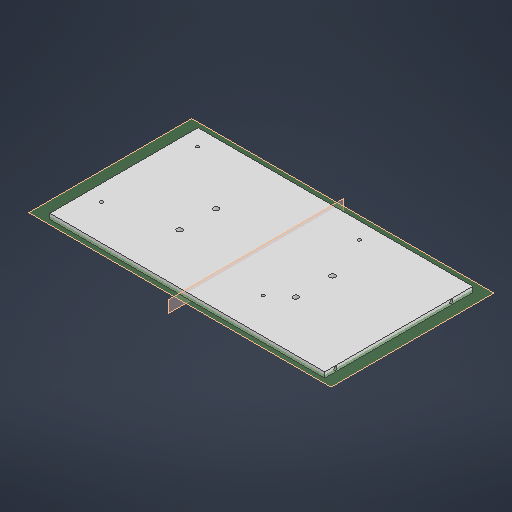
# Autodesk Inventor part: midplate
Saved by Autodesk Inventor 2025.1 (Build 291241000, 241)
## iProperties
Created: 2025-03-19
Part Number: midplate
Material: Generic
Document SubType Name: Modeling
Designer: m_kni
Density: 1 g/cm^3
Appearance: Default
Author: m_kni
Autodesk Inventor part; units mm, degrees
ref_plane "YZ Plane" through (0, 0, 0) normal (1, 0, 0) x (0, 1, 0)
ref_plane "XZ Plane" through (0, 0, 0) normal (0, 1, 0) x (-1, 0, 0)
ref_plane "XY Plane" through (0, 0, 0) normal (0, 0, 1) x (1, 0, 0)
sketch "Sketch1" plane through (0, 0, 0) normal (0, 1, 0) x (-1, 0, 0)
  circle A0 centre (-37.3734, -58.1709) radius 1.5
  circle A1 centre (112.6266, 30.8291) radius 1.5
  circle A2 centre (-37.3734, 30.8291) radius 1.5
  circle A3 centre (112.6266, -58.1709) radius 1.5
  circle A4 centre (54.1266, -16.9209) radius 2.5
  circle A5 centre (-53.8734, 17.0791) radius 2.5
  circle A6 centre (54.1266, 17.0791) radius 2.5
  circle A7 centre (-53.8734, -16.9209) radius 2.5
  line L0 (-127.3734, 73.8291) -> (127.6266, 73.8291)
  line L1 (-127.3734, -73.6709) -> (-127.3734, 73.8291)
  line L2 (127.6266, -73.6709) -> (-127.3734, -73.6709)
  line L3 (127.6266, 73.8291) -> (127.6266, -73.6709)
  point P0 (0, 0)
  point P1 (0.1266, 73.8291)
  constraints: 8 centre point, 8 end point
extrude "Extrusion1" add sketch "Sketch1" along normal blind 10
sketch "Sketch2" plane through (127.3734, 0, 73.8291) normal (1, 0, 0) x (0, 0, -1)
  line L0 (147.5, 0) -> (147.5, 10) projected
  line L1 (0, 0) -> (0, 10) projected
  circle A0 centre (127.5, 5) radius 1.5
  circle A1 centre (20, 5) radius 1.5
  point P0 (73.8291, 0)
  point P1 (0, 5)
  dimension "d2" = 20
  dimension "d3" = 20
  dimension "d4" = 3
  dimension "d5" = 3
  constraints: 2 centre point, 2 coincident, 1 midpoint
  measures "d2" distance from line of point (127.5, 5) L0
  measures "d3" distance of point (20, 5) point (0, 5)
  measures "d4" diameter of A0
  measures "d5" diameter of A1
extrude "Extrusion2" cut sketch "Sketch2" against normal blind 6
ref_plane "Work Plane1" through (-0.1266, 0, 73.8291) normal (1, 0, 0) x (0, 0, -1)
mirror "Mirror1" about plane through (-0.1266, 0, 73.8291) normal (1, 0, 0) of "Extrusion2"
sketch "Sketch3" plane through (-127.6266, 0, 73.8291) normal (0, 0, 1) x (1, 0, 0)
  line L0 (255, 10) -> (0, 10) projected
  line L1 (255, 0) -> (0, 0)
  line L2 (0, 0) -> (0, 10)
  line L3 (0, 10) -> (255, 10)
  line L4 (255, 10) -> (255, 0)
  point P0 (127.6266, 0)
  constraints: 8 end point, 2 parallel, 1 horizontal, 1 perpendicular
extrude "Extrusion3" cut sketch "Sketch3" against normal blind 10
sketch "Sketch4" plane through (0, 10, 0) normal (0, 1, 0) x (1, 0, 0)
  line L0 (127.3734, -63.8291) -> (127.3734, 73.6709) projected
  line L1 (-127.6266, -63.8291) -> (127.3734, -63.8291)
  line L2 (127.3734, -63.8291) -> (127.3734, 73.6709)
  line L3 (127.3734, 73.6709) -> (-127.6266, 73.6709)
  line L4 (-127.6266, 73.6709) -> (-127.6266, -63.8291)
  point P0 (0, 0)
  constraints: 8 end point, 2 parallel, 1 horizontal, 1 perpendicular
ref_plane "Work Plane2" through (0, 5, 0) normal (0, 1, 0) x (1, 0, 0)
extrude "Extrusion4" cut sketch "Sketch4" against normal blind 2.5
mirror "Mirror2" about plane through (0, 5, 0) normal (0, 1, 0) of "Extrusion4"
ref_plane "Work Plane3" through (0, 5, 0) normal (0, 1, 0) x (1, 0, 0)
body "Solid1"
